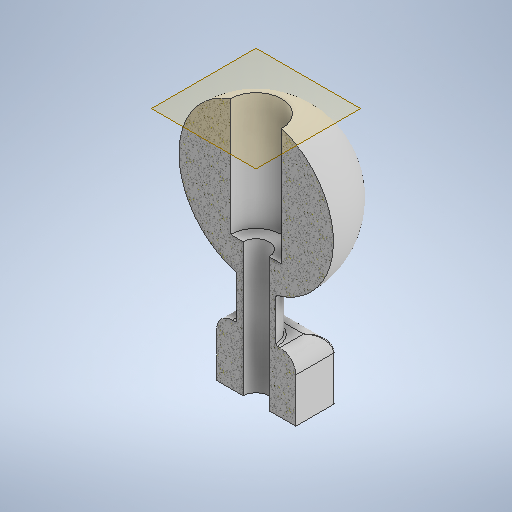
# Autodesk Inventor part: balljoint_male
Saved by Autodesk Inventor 2025.1 (Build 291241000, 241)
## iProperties
Created: 2024-10-31
Part Number: balljoint_male
Material: Generisch
Document SubType Name: Modeling
Designer: ZOMBULLI
Density: 1 g/cm^3
Appearance: Vorgabe
Author: ZOMBULLI
Autodesk Inventor part; units mm, degrees
ref_plane "YZ Plane" through (0, 0, 0) normal (1, 0, 0) x (0, 1, 0)
ref_plane "XZ Plane" through (0, 0, 0) normal (0, 1, 0) x (-1, 0, 0)
sketch "Skizze1" plane through (0, 0, 0) normal (0, 0, 1) x (1, 0, 0)
  circle A0 centre (0, 0) radius 2.5
  dimension "d0" = 5
  constraints: 1 centre point, 1 coincident
  measures "d0" diameter of A0
extrude "Extrusion1" add sketch "Skizze1" along normal blind 6
sketch "Skizze3" plane through (0, 0, 0) normal (0, 1, 0) x (-1, 0, 0)
  line L0 (0, 24.65) -> (0, 24.65)
  line L1 (0, 24.65) -> (0, 5.15)
  line L2 (0, 5.15) -> (0, 5.15)
  line L3 (9.75, 14.9) -> (9.75, 14.9)
  arc A0 (9.75, 14.9) -> (0, 24.65) centre (0, 14.9) ccw
  arc A1 (0, 5.15) -> (9.75, 14.9) centre (0, 14.9) ccw
  line L4 (2.5, 6) -> (-2.5, 6) projected
  line L5 (2.5, 0) -> (-2.5, 0) projected
  line L6 (0, -5.3339) -> (0, 32.0031) projected
  point P0 (0, 0)
  point P1 (9.75, 24.65)
  point P2 (0, 14.9)
  point P3 (0, 24.65)
  dimension "d6" = 19.5
  dimension "d7" = 9.75
  dimension "d8" = 9.75
  dimension "d10" = 14.9
  dimension "d11" = 0
  constraints: 8 end point, 4 point on circle, 4 tangent, 2 centre point, 2 parallel, 2 point on line, 1 concentric, 1 horizontal, 1 midpoint, 1 perpendicular
  measures "d6" distance of L0.end L1.end
  measures "d7" distance of point (9.75, 24.65) L0.end
  measures "d8" radius of A0
  measures "d10" distance from line of L5 A0.centre
  measures "d11" distance between parallel lines of L6 L1
revolve "Umdrehung1" add sketch "Skizze3" angle 360 about axis through (0, 0, 24.65) along (0, 0, -1)
ref_plane "Arbeitsebene1" through (0, 0, 24.65) normal (0, 0, 1) x (1, 0, 0)
sketch "Skizze6" plane through (0, 0, 0) normal (0, 0, -1) x (-1, 0, 0)
  line L0 (-5, -5) -> (5, -5)
  line L1 (5, -5) -> (5, 5)
  line L2 (5, 5) -> (-5, 5)
  line L3 (-5, 5) -> (-5, -5)
  point P0 (0, 0)
  dimension "d21" = 5
  dimension "d22" = 5
  dimension "d23" = 10
  dimension "d24" = 5
  constraints: 8 end point, 2 parallel, 1 horizontal, 1 perpendicular
  measures "d21" distance from line of L2 point (0, 0)
  measures "d22" distance from line of point (0, 0) L0
  measures "d23" distance between parallel lines of L1 L3
  measures "d24" distance from line of point (0, 0) L3
extrude "Extrusion5" add sketch "Skizze6" along normal blind 7.6
fillet "Rundung6" radius 2 4 edges at (0, -5, 0) (-5, 0, 0) (5, 0, 0) (0, 5, 0)
fillet "Rundung7" radius 0.2 1 edges at (-2.5, 0, 0)
fillet "Rundung8" radius 0.2 8 edges at (-4.4142, -4.4142, -0.5858) (-5, -5, -4.8) (-4.4142, 4.4142, -0.5858) (-5, 5, -4.8) (4.4142, -4.4142, -0.5858) (5, -5, -4.8) (4.4142, 4.4142, -0.5858) (5, 5, -4.8)
sketch "Skizze7" plane through (0, 0, 24.65) normal (0, 0, 1) x (1, 0, 0)
  circle A0 centre (0, 0) radius 1.65
  dimension "d33" = 3.3
  constraints: 1 centre point, 1 coincident
  measures "d33" diameter of A0
extrude "Extrusion6" cut sketch "Skizze7" against normal up to next
fillet "Rundung9" radius 0.2 2 edges at (0, -2.5, 5.476) (0, 2.5, 5.476)
sketch "Skizze8" plane through (0, 0, 24.65) normal (0, 0, 1) x (1, 0, 0)
  circle A0 centre (0, 0) radius 3.25
  dimension "d37" = 6.5
  constraints: 1 centre point, 1 coincident
  measures "d37" diameter of A0
extrude "Extrusion7" cut sketch "Skizze8" against normal blind 15.4
